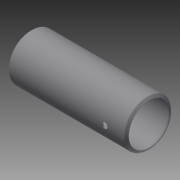
# Autodesk Inventor part: 04R-2.00453C
Saved by Autodesk Inventor 2014 SP2 (Build 180246200, 246)
## iProperties
Created: 2019-01-29
Part Number: 04R-2.00453C
Material: Generic
Catalog Web Link: www.cadenas.de
Description: Tube-Original Line - Standard Air Cylinders
Vendor: BIMBA
Document SubType Name: Modeling
Designer: psadmin
Manufacturer: BIMBA
Mass: 1.94099 g
Surface Area: 66.2968 cm^2
Volume: 1.94099 cm^3
Density: 1 g/cm^3
Appearance: PSOLRGB-180-180-180
Category: PARTsolutions
Company: BIMBA
Title: 04R-2.00453C
Author: Cadenas PARTsolutions
Comments: Original Line - Standard Air Cylinders
PSOL_IDENT_0: {$CADENAS_DATA\23d-libs\bimba\bimba\bimba_imperial\bimba_full_line\original_line_cylinders\standard_
PSOL_IDENT_1: air_cylinders\tube.prj},201 {VTYP=3D},{NB=04R-2.00453C},{LINA=04R-2.00453C},{NN=Tube},{DATE=21.03.20
PSOL_IDENT_2: 18 14:31:21},{GEOMDATE=18.02.2011 00:00:00},{VERSION=},{LINEID=40},{WBVAR=MNT,ACTING,NR,L,FOURHOLES,
PSOL_IDENT_3: SR},{WBNUMERIC=L,FOURHOLES}  {NB=04R-2.00453C},{LINA=04R-2.00453C},{KT=DUMMY},{PN=04R-2.00453C},{BOR
PSOL_IDENT_4: E=0.75000000},{BOREPN=04},{MNT=},{MNTALG='' , 'Front Nose' , 'BF' , 'Front Block' , 'BFT' , 'Front T
PSOL_IDENT_5: runnion' , 'A' , 'Adjustable Stroke'},{ACTING=R},{ACTINGALG= '' , 'Single Acting' , 'R' , 'Reverse/D
PSOL_IDENT_6: ouble Acting' },{NR=},{NRALG= '' , 'N/A' },{L=2.0045},{OD=0.8075},{ODN=0.8050},{ODP=0.8625},{ODB=0.8
PSOL_IDENT_7: 325},{ID=0.7615},{DV=0.00000000},{LV=0.00000000},{LV1=0.00000000},{G=0.0300},{FOURHOLES=3},{AA=0.375
PSOL_IDENT_8: 0},{BB=0.0940},{SR=C},{SRALG= 'C' , 'Carbon Steel Rod' , 'SR' , '303 Stainless Steel Rod' , '' , '30
PSOL_IDENT_9: 3 Stainless Steel Rod'}
NN: Tube
NT: Original Line - Standard Air Cylinders
NB: 04R-2.00453C
NBSYN: $PN.
LINA: 04R-2.00453C
BORE: 0
BOREPN: 04
MNT: Front Nose
MNTALG: '' , 'Front Nose' , 'BF' , 'Front Block' , 'BFT' , 'Front Trunnion' , 'A' , 'Adjustable Stroke'
ACTING: Reverse/Double Acting
NR: N/A
L: 2.0045
ODN: 0.805
ODP: 0.8625
ODB: 0.8325
ID: 0.7615
DV: 0
LV: 0
LV1: 0
G: 0.03
FOURHOLES: 3
AA: 0.375
BB: 0.094
SR: Carbon Steel Rod
SUPPLIER: BIMBA
ARTICLENO: 04R-2.00453C
BOMINFO: 04R-2.00453C
CREATOR: CADENAS GmbH
Autodesk Inventor part; units mm, degrees
sketch "Sketch_1" plane through (0, 0, 0) normal (0, 0, 1) x (1, 0, 0)
  line L0 (50.9143, 0) -> (0, 0)
  arc A0 (-0.6395, 9.3472) -> (-0.6395, 9.1676) centre (-0.5497, 9.2574) ccw
  line L1 (-0.6395, 9.1676) -> (-0.381, 8.9091)
  line L2 (-0.381, 8.9091) -> (0, 8.9091)
  line L3 (0, 8.9091) -> (0.762, 9.671)
  line L4 (0.762, 9.671) -> (50.1523, 9.671)
  line L5 (50.1523, 9.671) -> (50.9143, 8.9091)
  line L6 (50.9143, 8.9091) -> (51.2953, 8.9091)
  line L7 (51.2953, 8.9091) -> (51.5538, 9.1676)
  arc A1 (51.5538, 9.1676) -> (51.5538, 9.3472) centre (51.464, 9.2574) ccw
  line L8 (51.5538, 9.3472) -> (50.8689, 10.0321)
  arc A2 (50.8689, 10.0321) -> (50.3301, 10.2553) centre (50.3301, 9.4933) ccw
  line L9 (50.3301, 10.2553) -> (0.5842, 10.2553)
  arc A3 (0.5842, 10.2553) -> (0.0454, 10.0321) centre (0.5842, 9.4933) ccw
  line L10 (0.0454, 10.0321) -> (-0.6395, 9.3472)
  constraints: 22 end point, 8 point on circle, 4 centre point
revolve "Revolution1" add sketch "Sketch_1" angle 360 about axis through (50.9143, 0, 0) along (1, 0, 0)
sketch "Sketch_7" plane through (0, 0, 0) normal (0, 0, 1) x (1, 0, 0)
  circle A0 centre (42.1513, 0) radius 1.1938
  constraints: 1 centre point
extrude "Extrusion1" cut sketch "Sketch_7" along normal blind 10.2553
ref_plane "cp1_XY" through (25.4571, 10.2553, 0) normal (1, 0, 0) x (0, 0, -1)
ref_plane "cp1_YZ" through (25.4571, 10.2553, 0) normal (0, 0, -1) x (0, 1, 0)
ref_plane "cp1_ZX" through (25.4571, 10.2553, 0) normal (0, 1, 0) x (1, 0, 0)
ref_plane "cp2_XY" through (25.4571, 0, -10.2553) normal (1, 0, 0) x (0, 0, -1)
ref_plane "cp2_YZ" through (25.4571, 0, -10.2553) normal (0, 0, -1) x (0, 1, 0)
ref_plane "cp2_ZX" through (25.4571, 0, -10.2553) normal (0, 1, 0) x (1, 0, 0)
ref_plane "cp3_XY" through (25.4571, -10.2553, 0) normal (1, 0, 0) x (0, 0, -1)
ref_plane "cp3_YZ" through (25.4571, -10.2553, 0) normal (0, 0, -1) x (0, 1, 0)
ref_plane "cp3_ZX" through (25.4571, -10.2553, 0) normal (0, 1, 0) x (1, 0, 0)
ref_plane "cp4_XY" through (25.4571, 0, 10.2553) normal (1, 0, 0) x (0, 0, -1)
ref_plane "cp4_YZ" through (25.4571, 0, 10.2553) normal (0, 0, -1) x (0, 1, 0)
ref_plane "cp4_ZX" through (25.4571, 0, 10.2553) normal (0, 1, 0) x (1, 0, 0)
ref_plane "tube_front_XY" through (0, 0, 0) normal (1, 0, 0) x (0, 0, -1)
ref_plane "tube_front_YZ" through (0, 0, 0) normal (0, 0, -1) x (0, 1, 0)
ref_plane "tube_front_ZX" through (0, 0, 0) normal (0, 1, 0) x (1, 0, 0)
ref_plane "tube_rear_XY" through (50.9143, 0, 0) normal (1, 0, 0) x (0, 0, -1)
ref_plane "tube_rear_YZ" through (50.9143, 0, 0) normal (0, 0, -1) x (0, 1, 0)
ref_plane "tube_rear_ZX" through (50.9143, 0, 0) normal (0, 1, 0) x (1, 0, 0)
body "Solid1"
